Autodesk Inventor part; units mm, degrees
(part 2 of 2)
  spline S333 degree 2 poles (23.5178, 2.4138) (23.2926, 2.4138) (23.1418, 2.6467) knots 0 0 0 1 1 1
  spline S334 degree 2 poles (23.1418, 2.6467) (23.0114, 2.8062) (23.0114, 3.0478) knots 0 0 0 1 1 1
  spline S335 degree 2 poles (23.0114, 3.0478) (23.0114, 3.3426) (23.1476, 3.5185) knots 0 0 0 1 1 1
  spline S336 degree 2 poles (23.1476, 3.5185) (23.2858, 3.7002) (23.4975, 3.7002) knots 0 0 0 1 1 1
  spline S337 degree 2 poles (23.4975, 3.7002) (23.6454, 3.7002) (23.744, 3.6229) knots 0 0 0 1 1 1
  spline S338 degree 2 poles (23.744, 3.6229) (23.7894, 3.6007) (23.8522, 3.506) knots 0 0 0 1 1 1
  spline S339 degree 2 poles (23.8522, 3.506) (23.8696, 3.4808) (23.8696, 3.4509) knots 0 0 0 1 1 1
  spline S340 degree 2 poles (23.8696, 3.4509) (23.8696, 3.4141) (23.8136, 3.3629) (23.7778, 3.3629) knots 0 0 0 1 2 2 2
  spline S341 degree 2 poles (23.7778, 3.3629) (23.7304, 3.3629) (23.6966, 3.417) knots 0 0 0 1 1 1
  spline S342 degree 2 poles (23.6966, 3.417) (23.657, 3.4654) (23.6328, 3.4808) knots 0 0 0 1 1 1
  spline S343 degree 2 poles (23.6328, 3.4808) (23.5835, 3.5137) (23.4975, 3.5137) knots 0 0 0 1 1 1
  spline S344 degree 2 poles (23.4975, 3.5137) (23.3622, 3.5137) (23.195, 3.2595) (23.195, 3.0478) knots 0 0 0 1 2 2 2
  spline S345 degree 2 poles (23.195, 3.0478) (23.195, 2.8758) (23.28, 2.7444) knots 0 0 0 1 1 1
  spline S346 degree 2 poles (23.28, 2.7444) (23.3728, 2.6003) (23.5178, 2.6003) knots 0 0 0 1 1 1
  spline S347 degree 2 poles (23.5178, 2.6003) (23.6406, 2.6003) (23.6812, 2.726) knots 0 0 0 1 1 1
  spline S348 degree 2 poles (23.6812, 2.726) (23.7024, 2.7869) (23.7024, 2.9087) knots 0 0 0 1 1 1
  line L100 (23.7024, 2.9087) -> (23.5565, 2.9087)
  spline S349 degree 2 poles (23.5565, 2.9087) (23.4627, 2.9087) (23.4627, 3.0024) knots 0 0 0 1 1 1
  spline S350 degree 2 poles (23.4627, 3.0024) (23.4627, 3.0952) (23.5565, 3.0952) knots 0 0 0 1 1 1
  line L101 (23.5565, 3.0952) -> (23.8909, 3.0952)
  line L102 (23.8909, 3.0952) -> (23.8909, 2.8845)
  spline S351 degree 2 poles (25.1358, 2.5143) (25.1358, 2.4206) (25.0575, 2.4206) knots 0 0 0 1 1 1
  spline S352 degree 2 poles (25.0575, 2.4206) (25.0024, 2.4206) (24.9666, 2.4718) knots 0 0 0 1 1 1
  line L103 (24.9666, 2.4718) -> (24.3915, 3.3533)
  line L104 (24.3915, 3.3533) -> (24.3915, 2.5163)
  spline S353 degree 2 poles (24.3915, 2.5163) (24.3915, 2.4206) (24.2997, 2.4206) knots 0 0 0 1 1 1
  spline S354 degree 2 poles (24.2997, 2.4206) (24.2079, 2.4206) (24.2079, 2.5163) knots 0 0 0 1 1 1
  line L105 (24.2079, 2.5163) -> (24.2079, 3.6036)
  spline S355 degree 2 poles (24.2079, 3.6036) (24.2079, 3.6925) (24.293, 3.6925) knots 0 0 0 1 1 1
  spline S356 degree 2 poles (24.293, 3.6925) (24.349, 3.6925) (24.3886, 3.6364) knots 0 0 0 1 1 1
  line L106 (24.3886, 3.6364) -> (24.9521, 2.7782)
  line L107 (24.9521, 2.7782) -> (24.9521, 3.5978)
  spline S357 degree 2 poles (24.9521, 3.5978) (24.9521, 3.6925) (25.0439, 3.6925) knots 0 0 0 1 1 1
  spline S358 degree 2 poles (25.0439, 3.6925) (25.1358, 3.6925) (25.1358, 3.5978) knots 0 0 0 1 1 1
  line L108 (25.1358, 3.5978) -> (25.1358, 2.5143)
  spline S359 degree 2 poles (26.2579, 3.101) (26.2579, 2.7617) (26.0781, 2.5839) knots 0 0 0 1 1 1
  spline S360 degree 2 poles (26.0781, 2.5839) (25.9331, 2.4389) (25.7224, 2.4389) knots 0 0 0 1 1 1
  line L109 (25.7224, 2.4389) -> (25.3851, 2.4389)
  line L110 (25.3851, 2.4389) -> (25.3851, 3.6886)
  line L111 (25.3851, 3.6886) -> (25.7215, 3.6886)
  spline S361 degree 2 poles (25.7215, 3.6886) (25.9293, 3.6886) (26.08, 3.5514) knots 0 0 0 1 1 1
  spline S362 degree 2 poles (26.08, 3.5514) (26.2579, 3.388) (26.2579, 3.101) knots 0 0 0 1 1 1
  spline S363 degree 2 poles (26.0762, 3.101) (26.0762, 3.2972) (25.9583, 3.4064) knots 0 0 0 1 1 1
  spline S364 degree 2 poles (25.9583, 3.4064) (25.8568, 3.5002) (25.7205, 3.5002) knots 0 0 0 1 1 1
  line L112 (25.7205, 3.5002) -> (25.5668, 3.5002)
  line L113 (25.5668, 3.5002) -> (25.5668, 2.6255)
  line L114 (25.5668, 2.6255) -> (25.7224, 2.6255)
  spline S365 degree 2 poles (25.7224, 2.6255) (25.8616, 2.6255) (25.9544, 2.7105) knots 0 0 0 1 1 1
  spline S366 degree 2 poles (25.9544, 2.7105) (26.0762, 2.8565) (26.0762, 3.101) knots 0 0 0 1 1 1
  spline S367 degree 2 poles (21.3509, 15.2498) (21.3509, 14.9936) (21.2098, 14.868) knots 0 0 0 1 1 1
  spline S368 degree 2 poles (21.2098, 14.868) (21.1102, 14.7791) (20.9778, 14.7791) knots 0 0 0 1 1 1
  spline S369 degree 2 poles (20.9778, 14.7791) (20.7526, 14.7791) (20.6018, 15.012) knots 0 0 0 1 1 1
  spline S370 degree 2 poles (20.6018, 15.012) (20.4714, 15.1715) (20.4714, 15.4131) knots 0 0 0 1 1 1
  spline S371 degree 2 poles (20.4714, 15.4131) (20.4714, 15.7079) (20.6076, 15.8838) knots 0 0 0 1 1 1
  spline S372 degree 2 poles (20.6076, 15.8838) (20.7458, 16.0655) (20.9575, 16.0655) knots 0 0 0 1 1 1
  spline S373 degree 2 poles (20.9575, 16.0655) (21.1054, 16.0655) (21.204, 15.9882) knots 0 0 0 1 1 1
  spline S374 degree 2 poles (21.204, 15.9882) (21.2494, 15.9659) (21.3122, 15.8712) knots 0 0 0 1 1 1
  spline S375 degree 2 poles (21.3122, 15.8712) (21.3296, 15.8461) (21.3296, 15.8161) knots 0 0 0 1 1 1
  spline S376 degree 2 poles (21.3296, 15.8161) (21.3296, 15.7794) (21.2736, 15.7282) (21.2378, 15.7282) knots 0 0 0 1 2 2 2
  spline S377 degree 2 poles (21.2378, 15.7282) (21.1904, 15.7282) (21.1566, 15.7823) knots 0 0 0 1 1 1
  spline S378 degree 2 poles (21.1566, 15.7823) (21.117, 15.8306) (21.0928, 15.8461) knots 0 0 0 1 1 1
  spline S379 degree 2 poles (21.0928, 15.8461) (21.0435, 15.879) (20.9575, 15.879) knots 0 0 0 1 1 1
  spline S380 degree 2 poles (20.9575, 15.879) (20.8222, 15.879) (20.655, 15.6248) (20.655, 15.4131) knots 0 0 0 1 2 2 2
  spline S381 degree 2 poles (20.655, 15.4131) (20.655, 15.2411) (20.74, 15.1096) knots 0 0 0 1 1 1
  spline S382 degree 2 poles (20.74, 15.1096) (20.8328, 14.9656) (20.9778, 14.9656) knots 0 0 0 1 1 1
  spline S383 degree 2 poles (20.9778, 14.9656) (21.1006, 14.9656) (21.1412, 15.0913) knots 0 0 0 1 1 1
  spline S384 degree 2 poles (21.1412, 15.0913) (21.1624, 15.1521) (21.1624, 15.2739) knots 0 0 0 1 1 1
  line L115 (21.1624, 15.2739) -> (21.0165, 15.2739)
  spline S385 degree 2 poles (21.0165, 15.2739) (20.9227, 15.2739) (20.9227, 15.3677) knots 0 0 0 1 1 1
  spline S386 degree 2 poles (20.9227, 15.3677) (20.9227, 15.4605) (21.0165, 15.4605) knots 0 0 0 1 1 1
  line L116 (21.0165, 15.4605) -> (21.3509, 15.4605)
  line L117 (21.3509, 15.4605) -> (21.3509, 15.2498)
  spline S387 degree 2 poles (22.5958, 14.8796) (22.5958, 14.7858) (22.5175, 14.7858) knots 0 0 0 1 1 1
  spline S388 degree 2 poles (22.5175, 14.7858) (22.4624, 14.7858) (22.4266, 14.8371) knots 0 0 0 1 1 1
  line L118 (22.4266, 14.8371) -> (21.8515, 15.7185)
  line L119 (21.8515, 15.7185) -> (21.8515, 14.8815)
  spline S389 degree 2 poles (21.8515, 14.8815) (21.8515, 14.7858) (21.7597, 14.7858) knots 0 0 0 1 1 1
  spline S390 degree 2 poles (21.7597, 14.7858) (21.6679, 14.7858) (21.6679, 14.8815) knots 0 0 0 1 1 1
  line L120 (21.6679, 14.8815) -> (21.6679, 15.9688)
  spline S391 degree 2 poles (21.6679, 15.9688) (21.6679, 16.0578) (21.753, 16.0578) knots 0 0 0 1 1 1
  spline S392 degree 2 poles (21.753, 16.0578) (21.809, 16.0578) (21.8486, 16.0017) knots 0 0 0 1 1 1
  line L121 (21.8486, 16.0017) -> (22.4121, 15.1434)
  line L122 (22.4121, 15.1434) -> (22.4121, 15.963)
  spline S393 degree 2 poles (22.4121, 15.963) (22.4121, 16.0578) (22.5039, 16.0578) knots 0 0 0 1 1 1
  spline S394 degree 2 poles (22.5039, 16.0578) (22.5958, 16.0578) (22.5958, 15.963) knots 0 0 0 1 1 1
  line L123 (22.5958, 15.963) -> (22.5958, 14.8796)
  spline S395 degree 2 poles (23.7179, 15.4663) (23.7179, 15.127) (23.5381, 14.9492) knots 0 0 0 1 1 1
  spline S396 degree 2 poles (23.5381, 14.9492) (23.3931, 14.8042) (23.1824, 14.8042) knots 0 0 0 1 1 1
  line L124 (23.1824, 14.8042) -> (22.8451, 14.8042)
  line L125 (22.8451, 14.8042) -> (22.8451, 16.0539)
  line L126 (22.8451, 16.0539) -> (23.1815, 16.0539)
  spline S397 degree 2 poles (23.1815, 16.0539) (23.3893, 16.0539) (23.54, 15.9167) knots 0 0 0 1 1 1
  spline S398 degree 2 poles (23.54, 15.9167) (23.7179, 15.7533) (23.7179, 15.4663) knots 0 0 0 1 1 1
  spline S399 degree 2 poles (23.5362, 15.4663) (23.5362, 15.6625) (23.4183, 15.7717) knots 0 0 0 1 1 1
  spline S400 degree 2 poles (23.4183, 15.7717) (23.3168, 15.8654) (23.1805, 15.8654) knots 0 0 0 1 1 1
  line L127 (23.1805, 15.8654) -> (23.0268, 15.8654)
  line L128 (23.0268, 15.8654) -> (23.0268, 14.9907)
  line L129 (23.0268, 14.9907) -> (23.1824, 14.9907)
  spline S401 degree 2 poles (23.1824, 14.9907) (23.3216, 14.9907) (23.4144, 15.0758) knots 0 0 0 1 1 1
  spline S402 degree 2 poles (23.4144, 15.0758) (23.5362, 15.2217) (23.5362, 15.4663) knots 0 0 0 1 1 1
  line L130 (19.8219, 14.7791) -> (19.1395, 14.7791)
  spline S403 degree 2 poles (19.1395, 14.7791) (19.1704, 14.925) (19.2004, 15.0468) knots 0 0 0 1 1 1
  spline S404 degree 2 poles (19.2004, 15.0468) (19.2487, 15.2014) (19.3357, 15.3155) knots 0 0 0 1 1 1
  spline S405 degree 2 poles (19.3357, 15.3155) (19.4449, 15.4595) (19.6421, 15.5735) knots 0 0 0 1 1 1
  spline S406 degree 2 poles (19.6421, 15.5735) (19.7339, 15.6257) (19.7339, 15.7176) knots 0 0 0 1 1 1
  spline S407 degree 2 poles (19.7339, 15.7176) (19.7339, 15.7746) (19.6547, 15.8538) (19.587, 15.8538) knots 0 0 0 1 2 2 2
  spline S408 degree 2 poles (19.587, 15.8538) (19.5029, 15.8538) (19.4633, 15.8306) knots 0 0 0 1 1 1
  spline S409 degree 2 poles (19.4633, 15.8306) (19.4063, 15.7978) (19.3744, 15.7176) knots 0 0 0 1 1 1
  spline S410 degree 2 poles (19.3744, 15.7176) (19.3512, 15.6615) (19.2961, 15.6615) knots 0 0 0 1 1 1
  spline S411 degree 2 poles (19.2961, 15.6615) (19.2593, 15.6615) (19.2043, 15.7127) (19.2043, 15.7514) knots 0 0 0 1 2 2 2
  spline S412 degree 2 poles (19.2043, 15.7514) (19.2043, 15.7717) (19.212, 15.7891) knots 0 0 0 1 1 1
  spline S413 degree 2 poles (19.212, 15.7891) (19.3096, 16.0404) (19.5793, 16.0404) knots 0 0 0 1 1 1
  spline S414 degree 2 poles (19.5793, 16.0404) (19.7397, 16.0404) (19.8209, 15.9534) knots 0 0 0 1 1 1
  spline S415 degree 2 poles (19.8209, 15.9534) (19.9262, 15.8587) (19.9262, 15.7301) knots 0 0 0 1 1 1
  spline S416 degree 2 poles (19.9262, 15.7301) (19.9262, 15.5281) (19.5435, 15.302) (19.4565, 15.1657) knots 0 0 0 1 2 2 2
  spline S417 degree 2 poles (19.4565, 15.1657) (19.4034, 15.0826) (19.3686, 14.9656) knots 0 0 0 1 1 1
  line L131 (19.3686, 14.9656) -> (19.8219, 14.9656)
  spline S418 degree 2 poles (19.8219, 14.9656) (19.9137, 14.9656) (19.9137, 14.8728) knots 0 0 0 1 1 1
  spline S419 degree 2 poles (19.9137, 14.8728) (19.9137, 14.7791) (19.8219, 14.7791) knots 0 0 0 1 1 1
  spline S420 degree 2 poles (17.3795, 15.243) (17.3795, 15.0284) (17.2519, 14.898) knots 0 0 0 1 1 1
  spline S421 degree 2 poles (17.2519, 14.898) (17.1349, 14.7791) (16.9697, 14.7791) knots 0 0 0 1 1 1
  spline S422 degree 2 poles (16.9697, 14.7791) (16.8411, 14.7791) (16.7396, 14.8545) knots 0 0 0 1 1 1
  spline S423 degree 2 poles (16.7396, 14.8545) (16.6295, 14.9366) (16.584, 15.0787) knots 0 0 0 1 1 1
  spline S424 degree 2 poles (16.584, 15.0787) (16.5782, 15.099) (16.5782, 15.1154) knots 0 0 0 1 1 1
  spline S425 degree 2 poles (16.5782, 15.1154) (16.5782, 15.155) (16.6343, 15.2043) (16.6701, 15.2043) knots 0 0 0 1 2 2 2
  spline S426 degree 2 poles (16.6701, 15.2043) (16.7338, 15.2043) (16.7551, 15.1289) knots 0 0 0 1 1 1
  spline S427 degree 2 poles (16.7551, 15.1289) (16.7793, 15.0584) (16.8382, 15.0139) knots 0 0 0 1 1 1
  spline S428 degree 2 poles (16.8382, 15.0139) (16.8972, 14.9704) (16.9668, 14.9704) knots 0 0 0 1 1 1
  spline S429 degree 2 poles (16.9668, 14.9704) (17.0586, 14.9704) (17.1205, 15.0294) knots 0 0 0 1 1 1
  spline S430 degree 2 poles (17.1205, 15.0294) (17.1997, 15.1154) (17.1997, 15.242) knots 0 0 0 1 1 1
  spline S431 degree 2 poles (17.1997, 15.242) (17.1997, 15.3754) (17.1243, 15.4421) knots 0 0 0 1 1 1
  spline S432 degree 2 poles (17.1243, 15.4421) (17.0663, 15.4914) (16.9677, 15.5069) knots 0 0 0 1 1 1
  spline S433 degree 2 poles (16.9677, 15.5069) (16.9165, 15.5107) (16.8605, 15.5146) knots 0 0 0 1 1 1
  spline S434 degree 2 poles (16.8605, 15.5146) (16.8237, 15.5165) (16.7735, 15.5639) (16.7735, 15.5919) knots 0 0 0 1 2 2 2
  spline S435 degree 2 poles (16.7735, 15.5919) (16.7735, 15.6344) (16.8411, 15.6789) knots 0 0 0 1 1 1
  line L132 (16.8411, 15.6789) -> (17.0122, 15.8606)
  line L133 (17.0122, 15.8606) -> (16.7203, 15.8606)
  spline S436 degree 2 poles (16.7203, 15.8606) (16.6304, 15.8606) (16.6304, 15.9524) knots 0 0 0 1 1 1
  spline S437 degree 2 poles (16.6304, 15.9524) (16.6304, 16.0452) (16.7203, 16.0452) knots 0 0 0 1 1 1
  line L134 (16.7203, 16.0452) -> (17.2635, 16.0471)
  spline S438 degree 2 poles (17.2635, 16.0471) (17.3321, 16.0471) (17.3321, 15.992) knots 0 0 0 1 1 1
  spline S439 degree 2 poles (17.3321, 15.992) (17.3321, 15.9582) (17.25, 15.8799) knots 0 0 0 1 1 1
  line L135 (17.25, 15.8799) -> (17.0547, 15.6818)
  spline S440 degree 2 poles (17.0547, 15.6818) (17.3795, 15.6209) (17.3795, 15.243) knots 0 0 0 1 1 1
  line L136 (14.8124, 14.9714) -> (14.7322, 14.9714)
  line L137 (14.7322, 14.9714) -> (14.7322, 14.8728)
  spline S441 degree 2 poles (14.7322, 14.8728) (14.7322, 14.7791) (14.6404, 14.7791) knots 0 0 0 1 1 1
  spline S442 degree 2 poles (14.6404, 14.7791) (14.5486, 14.7791) (14.5486, 14.8728) knots 0 0 0 1 1 1
  line L138 (14.5486, 14.8728) -> (14.5486, 14.9714)
  line L139 (14.5486, 14.9714) -> (14.0498, 14.9714)
  spline S443 degree 2 poles (14.0498, 14.9714) (13.9812, 14.9714) (13.9812, 15.069) knots 0 0 0 1 1 1
  spline S444 degree 2 poles (13.9812, 15.069) (13.9812, 15.1058) (13.9947, 15.1473) knots 0 0 0 1 1 1
  line L140 (13.9947, 15.1473) -> (14.2866, 15.9872)
  spline S445 degree 2 poles (14.2866, 15.9872) (14.3089, 16.0491) (14.3707, 16.0491) knots 0 0 0 1 1 1
  spline S446 degree 2 poles (14.3707, 16.0491) (14.4084, 16.0491) (14.4703, 15.9959) (14.4703, 15.9582) knots 0 0 0 1 2 2 2
  spline S447 degree 2 poles (14.4703, 15.9582) (14.4703, 15.9408) (14.4625, 15.9254) knots 0 0 0 1 1 1
  line L141 (14.4625, 15.9254) -> (14.1929, 15.1579)
  line L142 (14.1929, 15.1579) -> (14.5486, 15.1579)
  line L143 (14.5486, 15.1579) -> (14.5486, 15.3483)
  spline S448 degree 2 poles (14.5486, 15.3483) (14.5486, 15.4411) (14.6404, 15.4411) knots 0 0 0 1 1 1
  spline S449 degree 2 poles (14.6404, 15.4411) (14.7322, 15.4411) (14.7322, 15.3483) knots 0 0 0 1 1 1
  line L144 (14.7322, 15.3483) -> (14.7322, 15.1579)
  line L145 (14.7322, 15.1579) -> (14.8134, 15.1579)
  spline S450 degree 2 poles (14.8134, 15.1579) (14.9062, 15.1579) (14.9062, 15.0652) knots 0 0 0 1 1 1
  spline S451 degree 2 poles (14.9062, 15.0652) (14.9062, 14.9714) (14.8124, 14.9714) knots 0 0 0 1 1 1
  point P0 (22.0392, 2.286)
  point P1 (24.638, 2.4138)
  point P2 (22.098, 14.7791)
  point P3 (19.558, 14.7791)
  point P4 (17.018, 14.7791)
  point P5 (14.478, 14.7791)
  dimension "d73" = 0
  dimension "d74" = 0.635
  dimension "d75" = 0
  dimension "d76" = 0
  dimension "d77" = 0.635
  dimension "d78" = 0.635
  dimension "d79" = 0.635
  constraints: 9 vertical alignment, 8 parallel, 7 horizontal alignment, 6 midpoint, 24 other
  measures "d73" angle of L4 L2
  measures "d74" distance of A0.centre L2.end
  measures "d75" horizontal distance of A2.centre L9.start
  measures "d76" horizontal distance of A3.centre L13.start
  measures "d77" distance of L20.start A4.centre
  measures "d78" vertical distance of A6.centre point (22.039, 2.286)
  measures "d79" distance from line of A8.centre L34
extrude "Extrusion14" add sketch "Sketch14" along normal blind 0.0254 contours S0 S1 S2 S3 S4 S5 S6 S7 S8 S9 S10 S11 S12 S13 S14 S15 S16 S17 S18 | S19 S20 S21 S22 S23 S24 S25 S26 S27 S28 S29 S30 S31 S32 S33 S34 S35 S36 S37 S38 S39 S40 S41 | S42 S43 L50 L51 S44 S45 L52 L53 S46 S47 L54 S48 S49 L55 L56 S50 S51 L57 | S52 S53 S54 S55 S56 S57 S58 S59 | S68 S69 S70 S71 S72 S73 S74 S75 S76 S77 S78 S79 S80 S81 S82 S83 S84 S85 S86 S87 S88 S89 S90 | S91 S92 L58 S93 S94 L59 | S95 S96 L60 L61 S97 S98 L62 L63 S99 S100 L64 S101 S102 L65 L66 S103 S104 L67 | S105 S106 L68 S107 S108 L69 | S109 S110 S111 S112 S113 S114 S115 S116 S117 S118 S119 S120 S121 S122 S123 S124 S125 S126 S127 S128 S129 S130 S131 | S132 S133 S134 S135 S136 S137 S138 S139 | S148 S149 S150 S151 S152 S153 S154 S155 S156 S157 S158 S159 S160 S161 S162 S163 S164 S165 S166 S167 S168 S169 S170 | S171 S172 S173 S174 S175 S176 S177 S178 S179 S180 S181 S182 S183 S184 S185 S186 S187 S188 S189 | S190 S191 S192 L70 L71 L72 S193 S194 L73 S195 S196 L74 L75 S197 S198 S199 L76 L77 | S200 S201 S202 S203 S204 S205 S206 S207 S208 S209 S210 S211 S212 S213 S214 S215 S216 S217 S218 S219 S220 S221 S222 | S223 S224 L78 L79 L80 S225 S226 | S231 S232 S233 L84 L85 L86 S234 S235 S236 L87 S237 S238 L88 | S239 S240 S241 S242 S243 S244 S245 S246 S247 S248 S249 S250 S251 S252 S253 S254 S255 S256 S257 S258 S259 S260 S261 | S262 S263 S264 S265 S266 S267 S268 S269 S270 S271 S272 S273 S274 S275 S276 S277 S278 S279 S280 | L92 L93 S281 S282 L94 L95 S283 S284 | L96 S285 S286 L97 S287 S288 S289 L98 L99 S290 S291 S292 | S293 S294 S295 S296 S297 S298 S299 S300 S301 S302 S303 S304 S305 S306 S307 S308 S309 S310 S311 | S312 S313 S314 S315 S316 S317 S318 S319 S320 S321 S322 S323 S324 S325 S326 S327 S328 S329 S330 | S331 S332 S333 S334 S335 S336 S337 S338 S339 S340 S341 S342 S343 S344 S345 S346 S347 S348 L100 S349 S350 L101 L102 | S351 S352 L103 L104 S353 S354 L105 S355 S356 L106 L107 S357 S358 L108 | S359 S360 L109 L110 L111 S361 S362 | S367 S368 S369 S370 S371 S372 S373 S374 S375 S376 S377 S378 S379 S380 S381 S382 S383 S384 L115 S385 S386 L116 L117 | S387 S388 L118 L119 S389 S390 L120 S391 S392 L121 L122 S393 S394 L123 | S395 S396 L124 L125 L126 S397 S398 | L130 S403 S404 S405 S406 S407 S408 S409 S410 S411 S412 S413 S414 S415 S416 S417 L131 S418 S419 | S420 S421 S422 S423 S424 S425 S426 S427 S428 S429 S430 S431 S432 S433 S434 S435 L132 L133 S436 S437 L134 S438 S439 L135 S440 | L136 L137 S441 S442 L138 L139 S443 S444 L140 S445 S446 S447 L141 L142 L143 S448 S449 L144 L145 S450 S451
equation "\"d77\" = d74"
equation "\"d78\" = d77"
equation "\"d79\" = d78"
body "Solid1"
